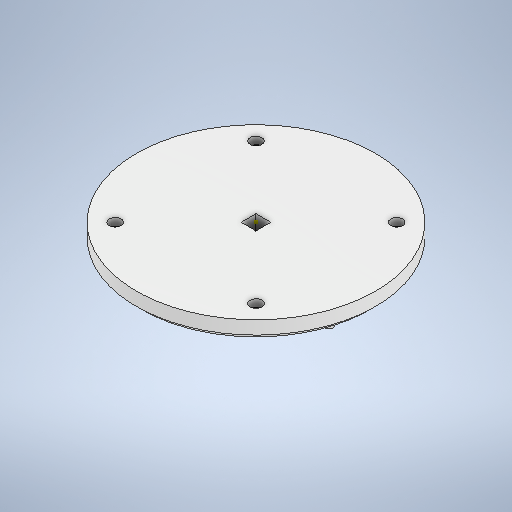
# Autodesk Inventor part: SCARA swivel base
Saved by Autodesk Inventor 2025.2 (Build 292293000, 293)
## iProperties
Created: 2025-01-25
Part Number: SCARA swivel base
Material: Generic
Document SubType Name: Modeling
Designer: caomi
Density: 1 g/cm^3
Appearance: Default
Author: caomi
Autodesk Inventor part; units mm, degrees
ref_plane "YZ Plane" through (0, 0, 0) normal (1, 0, 0) x (0, 1, 0)
ref_plane "XZ Plane" through (0, 0, 0) normal (0, 1, 0) x (-1, 0, 0)
ref_plane "XY Plane" through (0, 0, 0) normal (0, 0, 1) x (1, 0, 0)
sketch "Sketch1" plane through (0, 0, 0) normal (1, 0, 0) x (0, 1, 0)
  line L0 (0, 0) -> (0, -17.5)
  line L1 (15, -45) -> (22, -45)
  line L2 (22, -45) -> (22, 0)
  line L3 (22, 0) -> (0, 0)
  line L4 (0, -17.5) -> (15, -17.5)
  line L5 (15, -17.5) -> (15, -45)
  dimension "d2" = 17.5
  dimension "d3" = 45
  dimension "d4" = 22
  dimension "d11" = 15
  constraints: 12 end point, 3 vertical, 2 horizontal, 1 perpendicular
  measures "d2" distance of L0.end L0.start
  measures "d3" vertical distance of L1.start L0.start
  measures "d4" distance of L2.end L0.start
  measures "d11" distance of L0.end L4.end
revolve "Revolution1" add sketch "Sketch1" angle 360 about axis through (0, 22, 0) along (0, -1, 0)
sketch "Sketch2" plane through (0, 22, 0) normal (0, 1, 0) x (1, 0, 0)
  line L0 (2.8, -2.8) -> (-2.8, -2.8)
  line L1 (-2.8, -2.8) -> (-2.8, 2.8)
  line L2 (-2.8, 2.8) -> (2.8, 2.8)
  line L3 (2.8, 2.8) -> (2.8, -2.8)
  line L4 (2.8, -2.8) -> (-2.8, 2.8) construction
  line L5 (-2.8, -2.8) -> (2.8, 2.8) construction
  point P0 (0, 0)
  point P1 (0, 0)
  dimension "d7" = 5.6
  constraints: 12 end point, 2 parallel, 2 perpendicular, 1 coincident, 1 horizontal, 1 midpoint
  measures "d7" distance of L0.end L1.end
extrude "Extrusion1" cut sketch "Sketch2" against normal up to surface (22 mm away)
sketch "Sketch3" plane through (0, 0, 0) normal (1, 0, 0) x (0, 1, 0)
  point P0 (0, 0)
sketch "Sketch4" plane through (0, 0, 0) normal (1, 0, 0) x (0, 1, 0)
  line L0 (10.8004, 31.8094) -> (6.0445, 15.8122)
  line L1 (10.8004, 31.8094) -> (15.5479, 31.8094)
  point P0 (0, 0)
  constraints: 4 end point, 1 horizontal
extrude "Rib1" add sketch "Sketch4" along normal mid plane 3 rib yes fills toward (13.1742, 31.7594) open curves L1 L0
pattern_circular "Circular Pattern1" count 6 over 360 about axis through (0, 7.5, 0) along (0, -1, 0) of "Rib1"
sketch "Sketch5" plane through (0, 0, 0) normal (0, -1, 0) x (1, 0, 0)
  line L0 (17.4356, 1.5) -> (27.4356, 1.5)
  circle A0 centre (0, 0) radius 17.5 projected
  line L1 (17.4356, -1.5) -> (27.4356, -1.5)
  line L2 (-3.235, 0) -> (43.5251, 0) construction
  circle A1 centre (27.4356, 0) radius 1.5
  circle A2 centre (0, 0) radius 17.5
  point P0 (0, 0)
  point P1 (22.4356, -1.5)
  dimension "d21" = 3
  dimension "d22" = 10
  constraints: 6 end point, 4 point on circle, 3 horizontal, 2 centre point, 2 point on line, 1 coincident, 1 midpoint, 1 tangent, 1 other
  measures "d21" distance from line of point (22.436, -1.5) L0
  measures "d22" distance of L1.start L1.end
extrude "Extrusion2" add sketch "Sketch5" against normal up to surface (15 mm away) contours L0 A1 L1 A0 | A1
sketch "Sketch6" plane through (0, 22, 0) normal (0, 1, 0) x (1, 0, 0)
  point P0 (0, 0)
extrude "Extrusion3" cut sketch "Sketch5" against normal blind 2 contours L0 A1 L1 A0 | A1
sketch "Sketch7" plane through (0, 15, 0) normal (0, -1, 0) x (1, 0, 0)
  line L0 (26.5165, -26.5165) -> (0, 0) construction
  line L1 (0, 0) -> (26.7562, 0) construction
  dimension "d34" = 37.5
  dimension "d42" = 45
  constraints: 4 end point, 1 horizontal
  measures "d34" distance of L0.start L0.end
  measures "d42" angle of L0 L1
hole "Hole1" at (26.5165, 15, -26.5165) direction (0, 1, 0) diameter 4.5 end through all counterbore diameter 7.5 counterbore depth 4.2
pattern_circular "Circular Pattern2" count 4 over 360 about axis through (0, 18.5, 0) along (0, -1, 0) of "Hole1"
chamfer "Chamfer1" distance 2 angle 45 1 edges at (0, 15, 45)
body "Solid1"
